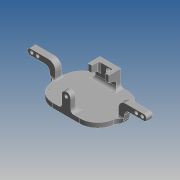
# Autodesk Inventor part: I006
Saved by Autodesk Inventor 2017 (Build 210142000, 142)
## iProperties
Created: 2018-10-19
Part Number: I006
Material: Générique
Document SubType Name: Modeling
Designer: Gilles Mottiez
Density: 1 g/cm^3
Appearance: Par défaut
Description: Plateforme mobile
Author: Gilles Mottiez
Autodesk Inventor part; units mm, degrees
ref_plane "YZ Plane" through (0, 0, 0) normal (1, 0, 0) x (0, 1, 0)
ref_plane "XZ Plane" through (0, 0, 0) normal (0, 1, 0) x (-1, 0, 0)
ref_plane "XY Plane" through (0, 0, 0) normal (0, 0, 1) x (1, 0, 0)
sketch "Sketch1" plane through (0, 0, 0) normal (0, 0, 1) x (1, 0, 0)
  line L0 (0, 0) -> (106, 0)
  line L1 (106, 0) -> (106, -80)
  line L2 (106, -80) -> (0, -80)
  line L3 (0, -80) -> (0, 0)
  dimension "d0" = 106
  dimension "d1" = 80
  constraints: 8 end point, 2 parallel, 1 horizontal, 1 perpendicular
  measures "d0" distance of L0.start L0.end
  measures "d1" distance of L2.end L0.start
extrude "Extrusion1" add sketch "Sketch1" along normal blind 8
sketch "Esquisse2" plane through (0, 0, 8) normal (0, 0, 1) x (1, 0, 0)
  line L0 (106, 0) -> (0, 0) construction
  line L1 (0, 0) -> (0, -80) construction
  line L2 (0, -80) -> (106, -80) construction
  line L3 (106, -80) -> (106, 0) construction
  line L4 (8, -15.5) -> (66, -15.5) construction
  line L5 (66, -15.5) -> (66, -64.5) construction
  line L6 (66, -64.5) -> (8, -64.5) construction
  line L7 (8, -64.5) -> (8, -15.5) construction
  line L8 (0, -40) -> (106, -40) construction
  dimension "d4" = 58
  dimension "d5" = 49
  dimension "d6" = 8
  constraints: 10 end point, 4 coincident, 2 midpoint, 2 parallel, 1 horizontal, 1 perpendicular, 1 other
  measures "d4" distance of L4.start L4.end
  measures "d5" distance of L4.end L5.end
  measures "d6" distance between parallel lines of L1 L7
hole "Perçage1" at (8, -15.5, 8) at (8, -64.5, 8) at (66, -64.5, 8) at (66, -15.5, 8) direction (0, 0, -1) diameter 2 end through all
sketch "Esquisse3" plane through (106, -80, 0) normal (1, 0, 0) x (0, 0, -1)
  line L0 (0, 80) -> (0, 0) construction
  line L1 (0, 80) -> (-8, 80) construction
  line L2 (-8, 0) -> (-8, 80) construction
  line L3 (0, 0) -> (-8, 0) construction
  line L4 (-8, 40) -> (0, 40) construction
  line L5 (0, 45) -> (-33, 45)
  line L6 (-33, 45) -> (-33, 35)
  line L7 (-33, 35) -> (0, 35)
  line L8 (0, 35) -> (0, 45)
  dimension "d14" = 33
  dimension "d15" = 10
  constraints: 10 end point, 2 midpoint, 2 parallel, 1 horizontal, 1 perpendicular, 1 point on line, 1 other
  measures "d14" distance of L7.end L6.end
  measures "d15" distance of L5.end L6.end
extrude "Extrusion2" add sketch "Esquisse3" along normal blind 10
sketch "Esquisse4" plane through (0, -80, 0) normal (-1, 0, 0) x (0, 0, 1)
  line L0 (0, 0) -> (0, 80) construction
  line L1 (0, 0) -> (8, 0) construction
  line L2 (8, 80) -> (8, 0) construction
  line L3 (0, 80) -> (8, 80) construction
  line L4 (8, 40) -> (0, 40) construction
  line L5 (0, 45) -> (33, 45)
  line L6 (33, 45) -> (33, 35)
  line L7 (33, 35) -> (0, 35)
  line L8 (0, 35) -> (0, 45)
  dimension "d18" = 33
  dimension "d19" = 10
  constraints: 10 end point, 2 midpoint, 2 parallel, 1 horizontal, 1 perpendicular, 1 point on line, 1 other
  measures "d18" distance of L6.end L7.end
  measures "d19" distance of L5.end L6.end
extrude "Extrusion3" add sketch "Esquisse4" along normal blind 10
sketch "Esquisse5" plane through (-10, -80, 0) normal (-1, 0, 0) x (0, 0, 1)
  line L0 (33, 45) -> (0, 45) construction
  line L1 (0, 45) -> (0, 35) construction
  line L2 (0, 35) -> (33, 35) construction
  line L3 (33, 35) -> (33, 45) construction
  line L4 (33, 45) -> (23, 45)
  line L5 (23, 45) -> (23, 35)
  line L6 (23, 35) -> (33, 35)
  line L7 (33, 35) -> (33, 45)
  point P0 (0, 80)
  dimension "d22" = 10
  constraints: 8 end point, 2 parallel, 1 horizontal, 1 perpendicular, 1 point on line
  measures "d22" distance of L6.end L5.end
extrude "Extrusion4" add sketch "Esquisse5" along normal blind 37.5
sketch "Esquisse6" plane through (116, -80, 0) normal (1, 0, 0) x (0, 0, -1)
  line L0 (0, 45) -> (-33, 45) construction
  line L1 (-33, 45) -> (-33, 35) construction
  line L2 (-33, 35) -> (0, 35) construction
  line L3 (0, 35) -> (0, 45) construction
  line L4 (-33, 35) -> (-23, 35)
  line L5 (-23, 35) -> (-23, 45)
  line L6 (-23, 45) -> (-33, 45)
  line L7 (-33, 45) -> (-33, 35)
  point P0 (0, 80)
  dimension "d25" = 10
  constraints: 8 end point, 2 parallel, 1 horizontal, 1 perpendicular, 1 point on line
  measures "d25" distance of L6.end L5.end
extrude "Extrusion5" add sketch "Esquisse6" along normal blind 37.5
sketch "Esquisse7" plane through (0, -80, 0) normal (0, -1, 0) x (1, 0, 0)
  line L0 (106, 0) -> (0, 0) construction
  line L1 (106, 0) -> (106, 8) construction
  line L2 (0, 8) -> (106, 8) construction
  line L3 (0, 0) -> (0, 8) construction
  line L4 (53, 8) -> (53, 0) construction
  line L5 (45.5, 8) -> (60.5, 8) construction
  line L6 (60.5, 8) -> (60.5, 28) construction
  line L7 (60.5, 28) -> (45.5, 28) construction
  line L8 (45.5, 28) -> (45.5, 8) construction
  circle A0 centre (53, 28) radius 7.5 construction
  arc A1 (60.5, 28) -> (45.5, 28) centre (53, 28) ccw
  line L9 (45.5, 28) -> (45.5, 8)
  line L10 (60.5, 28) -> (60.5, 8)
  line L11 (45.5, 8) -> (60.5, 8)
  circle A2 centre (53, 28) radius 2.5
  point P0 (0, 0)
  dimension "d28" = 15
  dimension "d29" = 20
  dimension "d30" = 5
  constraints: 16 end point, 4 tangent, 3 collinear, 3 midpoint, 2 centre point, 2 parallel, 2 point on circle, 2 vertical, 1 coincident, 1 horizontal, 1 horizontal alignment, 1 perpendicular, 1 point on line, 3 other
  measures "d28" distance of L7.end L6.end
  measures "d29" distance of L6.end L5.end
  measures "d30" diameter of A2
extrude "Extrusion6" add sketch "Esquisse7" against normal blind 8
sketch "Esquisse8" plane through (0, 0, 0) normal (0, 1, 0) x (1, 0, 0)
  line L0 (0, 0) -> (106, 0) construction
  line L1 (0, 0) -> (0, -8) construction
  line L2 (106, -8) -> (0, -8) construction
  line L3 (106, 0) -> (106, -8) construction
  line L4 (53, -8) -> (53, 0) construction
  line L5 (64.8, -8) -> (29.8, -8) construction
  line L6 (29.8, -8) -> (29.8, -35) construction
  line L7 (29.8, -35) -> (64.8, -35) construction
  line L8 (64.8, -35) -> (64.8, -8) construction
  circle A0 centre (53, -28) radius 2.5 construction
  line L9 (45.5, -8) -> (45.5, -28) construction
  arc A1 (45.5, -28) -> (60.5, -28) centre (53, -28) ccw construction
  line L10 (60.5, -28) -> (60.5, -8) construction
  line L11 (45.5, -8) -> (60.5, -8) construction
  line L12 (58.8, -35) -> (35.8, -35) construction
  line L13 (35.8, -35) -> (35.8, -23) construction
  line L14 (35.8, -23) -> (58.8, -23) construction
  line L15 (58.8, -23) -> (58.8, -35) construction
  line L16 (47.3, -23) -> (47.3, -35) construction
  line L17 (64.8, -35) -> (29.8, -35)
  line L18 (29.8, -35) -> (29.8, -8)
  line L19 (29.8, -8) -> (64.8, -8)
  line L20 (64.8, -8) -> (64.8, -35)
  circle A2 centre (53, -28) radius 5
  dimension "d33" = 27
  dimension "d34" = 35
  dimension "d35" = 23
  dimension "d36" = 12
  dimension "d37" = 5.8
  dimension "d38" = 10
  constraints: 28 end point, 6 parallel, 4 midpoint, 3 horizontal, 3 perpendicular, 2 point on line, 1 centre point, 1 coincident, 1 other
  measures "d33" distance of L5.end L6.end
  measures "d34" distance of L6.end L7.end
  measures "d35" distance of L13.end L14.end
  measures "d36" distance of L12.end L13.end
  measures "d37" distance from line of A0.centre L15
  measures "d38" diameter of A2
extrude "Extrusion7" add sketch "Esquisse8" against normal blind 8
sketch "Esquisse9" plane through (0, -8, 0) normal (0, -1, 0) x (1, 0, 0)
  circle A0 centre (53, 28) radius 5 construction
  line L0 (0, 0) -> (106, 0) construction
  line L1 (0, 0) -> (0, 8) construction
  line L2 (29.8, 8) -> (0, 8) construction
  line L3 (29.8, 8) -> (29.8, 35) construction
  line L4 (29.8, 35) -> (64.8, 35) construction
  line L5 (64.8, 35) -> (64.8, 8) construction
  line L6 (106, 8) -> (64.8, 8) construction
  line L7 (106, 0) -> (106, 8) construction
  line L8 (53, 28) -> (29.8, 28) construction
  line L9 (36.2, 22) -> (29.8, 22) construction
  line L10 (29.8, 22) -> (29.8, 34) construction
  line L11 (29.8, 34) -> (36.2, 34) construction
  line L12 (36.2, 34) -> (36.2, 22) construction
  line L13 (64.8, 34) -> (59.2, 34) construction
  line L14 (59.2, 34) -> (59.2, 22) construction
  line L15 (59.2, 22) -> (64.8, 22) construction
  line L16 (64.8, 22) -> (64.8, 34) construction
  line L17 (29.8, 34) -> (36.2, 34) construction
  line L18 (36.2, 34) -> (36.2, 22) construction
  line L19 (36.2, 22) -> (29.8, 22) construction
  line L20 (29.8, 22) -> (29.8, 34) construction
  line L21 (59.2, 34) -> (64.8, 34) construction
  line L22 (64.8, 34) -> (64.8, 22) construction
  line L23 (64.8, 22) -> (59.2, 22) construction
  line L24 (59.2, 22) -> (59.2, 34) construction
  line L25 (29.8, 35) -> (36.2, 35)
  line L26 (36.2, 35) -> (36.2, 22)
  line L27 (36.2, 22) -> (29.8, 22)
  line L28 (29.8, 22) -> (29.8, 35)
  line L29 (64.8, 35) -> (59.2, 35)
  line L30 (59.2, 35) -> (59.2, 22)
  line L31 (59.2, 22) -> (64.8, 22)
  line L32 (64.8, 22) -> (64.8, 35)
  dimension "d41" = 12
  dimension "d42" = 23
  dimension "d43" = 6.2
  constraints: 50 end point, 12 parallel, 7 perpendicular, 6 horizontal, 3 point on line, 2 horizontal alignment, 1 other
  measures "d41" distance of L11.end L9.start
  measures "d42" distance between parallel lines of L12 L14
  measures "d43" distance from line of L8.start L14
extrude "Extrusion8" add sketch "Esquisse9" along normal blind 12
sketch "Esquisse10" plane through (106, -45, 8) normal (0, -1, 0) x (1, 0, 0)
  line L0 (0, 25) -> (0, 0) construction
  line L1 (0, -8) -> (0, 0) construction
  line L2 (0, -8) -> (10, -8) construction
  line L3 (10, 15) -> (10, -8) construction
  line L4 (10, 15) -> (47.5, 15) construction
  line L5 (47.5, 25) -> (47.5, 15) construction
  line L6 (0, 25) -> (47.5, 25) construction
  line L7 (47.5, 20) -> (0, 20) construction
  circle A0 centre (40, 20) radius 2.5
  circle A1 centre (30, 20) radius 2.5
  point P0 (-106, -8)
  dimension "d46" = 7.5
  dimension "d47" = 10
  dimension "d48" = 5
  dimension "d49" = 5
  constraints: 3 point on line, 2 centre point, 2 coincident, 2 end point, 1 midpoint, 1 parallel
  measures "d46" distance from line of L5 point (40, 20)
  measures "d47" distance of point (30, 20) point (40, 20)
  measures "d48" diameter of A0
  measures "d49" diameter of A1
extrude "Extrusion9" cut sketch "Esquisse10" against normal through all
sketch "Esquisse11" plane through (0, -45, 8) normal (0, -1, 0) x (1, 0, 0)
  line L0 (0, 25) -> (0, 0) construction
  line L1 (0, 25) -> (-47.5, 25) construction
  line L2 (-47.5, 15) -> (-47.5, 25) construction
  line L3 (-10, 15) -> (-47.5, 15) construction
  line L4 (-10, -8) -> (-10, 15) construction
  line L5 (0, -8) -> (-10, -8) construction
  line L6 (0, 0) -> (0, -8) construction
  line L7 (-47.5, 20) -> (0, 20) construction
  circle A0 centre (-40, 20) radius 2.5
  circle A1 centre (-30, 20) radius 2.5
  point P0 (0, -8)
  dimension "d52" = 5
  dimension "d53" = 5
  dimension "d54" = 7.5
  dimension "d55" = 10
  constraints: 3 point on line, 2 centre point, 2 end point, 1 midpoint, 1 perpendicular
  measures "d52" diameter of A0
  measures "d53" diameter of A1
  measures "d54" distance from line of L2 A0.centre
  measures "d55" distance of A1.centre A0.centre
extrude "Extrusion10" cut sketch "Esquisse11" against normal through all
fillet "Congé1" radius 5 4 edges at (153.5, -40, 33) (153.5, -40, 23) (-47.5, -40, 33) (-47.5, -40, 23)
sketch "Esquisse12" plane through (0, 0, 8) normal (0, 0, 1) x (1, 0, 0)
  line L0 (106, -35) -> (106, 0) construction
  line L1 (106, 0) -> (64.8, 0) construction
  line L2 (64.8, 0) -> (64.8, -8) construction
  line L3 (64.8, -8) -> (29.8, -8) construction
  line L4 (29.8, -8) -> (29.8, 0) construction
  line L5 (29.8, 0) -> (0, 0) construction
  line L6 (0, -45) -> (0, -80) construction
  line L7 (0, -80) -> (45.5, -80) construction
  line L8 (45.5, -80) -> (45.5, -72) construction
  line L9 (45.5, -72) -> (60.5, -72) construction
  line L10 (60.5, -72) -> (60.5, -80) construction
  line L11 (60.5, -80) -> (106, -80) construction
  circle A0 centre (66, -15.5) radius 1 construction
  circle A1 centre (8, -64.5) radius 1 construction
  circle A2 centre (8, -15.5) radius 1 construction
  circle A3 centre (66, -64.5) radius 1 construction
  line L12 (0, -35) -> (0, -45) construction
  line L13 (0, 0) -> (106, 0) construction
  line L14 (0, -35) -> (0, -45) projected
  line L15 (106, -45) -> (106, -35) projected
  line L16 (0, 0) -> (0, -35) projected
  line L17 (106, -80) -> (106, -45) projected
  point P0 (53, -40)
  point P1 (0, -40)
  point P2 (53, 0)
  constraints: 2 midpoint, 1 horizontal alignment, 1 vertical alignment
ref_plane "Plan de construction1" through (53, -40, 8) normal (0, 1, 0) x (1, 0, 0)
fillet "Congé5" radius 30 4 edges at (0, 0, 4) (0, -80, 4) (106, -80, 4) (106, 0, 4)
fillet "Congé6" radius 2 2 edges at (0, -40, 8) (106, -40, 8)
fillet "Congé7" radius 10 4 edges at (0, -45, 4) (0, -35, 4) (106, -45, 4) (106, -35, 4)
fillet "Congé8" radius 2 4 edges at (109.8431, -35, 8) (109.8431, -45, 8) (-3.8431, -45, 8) (-3.8431, -35, 8)
fillet "Congé9" radius 5 4 edges at (60.5, -76, 8) (45.5, -76, 8) (64.8, -4, 8) (29.8, -4.0003, 8)
fillet "Congé10" radius 5 6 edges at (27.3, -8, 8) (47.3, -8, 8) (67.3, -8, 8) (43, -72, 8) (53, -72, 8) (63, -72, 8)
fillet "Congé11" radius 8 2 edges at (-10, -40, 23) (116, -40, 23)
fillet "Congé12" radius 3 2 edges at (33, -8, 22) (62, -8, 22)
fillet "Congé13" radius 3 2 edges at (36.2, -8, 20.5) (36.2, -8, 28.5)
fillet "Congé14" radius 1 2 edges at (59.2, -8, 28.5) (59.2, -8, 20.5)
fillet "Congé17" radius 12 2 edges at (0, -40, 33) (106, -40, 33)
chamfer "Chanfrein8" distance 2 distance2 9 1 edges at (33, -20, 22) measured on face at (33, -20, 22.5)
chamfer "Chanfrein9" distance 2 distance2 9 1 edges at (62, -20, 22) measured on face at (62, -20, 22.5)
chamfer "Chanfrein10" distance 15 distance2 3 1 edges at (-10, -40, 0) measured on face at (-10, -40, 0.5)
chamfer "Chanfrein11" distance 15 distance2 3 1 edges at (116, -40, 0) measured on face at (116, -40, 0.5)
fillet "Congé18" radius 7 2 edges at (-7, -40, 0) (113, -40, 0)
